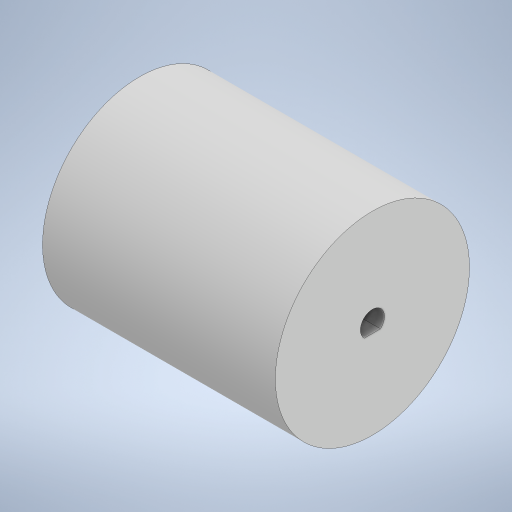
# Autodesk Inventor part: kolo
Saved by Autodesk Inventor 2023 (Build 270158000, 158)
## iProperties
Created: 2024-04-04
Part Number: kolo
Material: Ogólny
Document SubType Name: Modeling
Designer: Kamil
Density: 1 g/cm^3
Appearance: Domyślna
Author: Kamil
Autodesk Inventor part; units mm, degrees
ref_plane "YZ Plane" through (0, 0, 0) normal (1, 0, 0) x (0, 1, 0)
ref_plane "XZ Plane" through (0, 0, 0) normal (0, 1, 0) x (-1, 0, 0)
ref_plane "XY Plane" through (0, 0, 0) normal (0, 0, 1) x (1, 0, 0)
sketch "Szkic1" plane through (0, 0, 0) normal (1, 0, 0) x (0, 1, 0)
  circle A0 centre (0, 0) radius 12.5
  dimension "d0" = 25
  constraints: 1 centre point, 1 coincident
  measures "d0" diameter of A0
extrude "Wyciągnięcie proste1" add sketch "Szkic1" along normal blind 30
sketch "Szkic2" plane through (0, 0, 0) normal (-1, 0, 0) x (0, 0, 1)
  circle A0 centre (0, 0) radius 1.55
  dimension "d3" = 3.1
  constraints: 1 centre point, 1 coincident
  measures "d3" diameter of A0
extrude "Wyciągnięcie proste2" cut sketch "Szkic2" against normal blind 30
sketch "Szkic4" plane through (0, 0, 0) normal (-1, 0, 0) x (0, 0, 1)
  circle A0 centre (0, 0) radius 12.5 projected
  circle A1 centre (0, 0) radius 8.5
  dimension "d6" = 4
  constraints: 1 centre point
  measures "d6" radial gap between concentric circles of A0 A1
extrude "Wyciągnięcie proste3" cut sketch "Szkic4" against normal blind 15 contours A1
sketch "Szkic5" plane through (15, 0, 0) normal (-1, 0, 0) x (0, 0, 1)
  circle A0 centre (0, 0) radius 1.55 projected
  circle A1 centre (0, 0) radius 1.55 projected
  line L0 (-1.0392, -1.15) -> (1.0392, -1.15)
  point P0 (0, -1.15)
  point P1 (1.0392, -1.15)
  point P2 (-1.0392, -1.15)
  dimension "d9" = 1.15
  constraints: 2 end point, 2 point on circle, 1 horizontal, 1 midpoint
  measures "d9" distance of point (0, -1.15) point (0, 0)
extrude "Wyciągnięcie proste4" add sketch "Szkic5" against normal up to surface (15 mm away) contours L0 A0 picked at (-0.2431, -1.2226)
